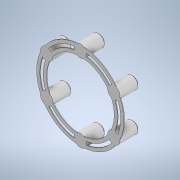
# Autodesk Inventor part: СкреплениеКатков
Saved by Autodesk Inventor 2020 (Build 240168000, 168)
## iProperties
Created: 2021-03-14
Part Number: СкреплениеКатков
Material: Типовые
Document SubType Name: Modeling
Designer: I_Love_U_Bogdan
Density: 1 g/cm^3
Appearance: По умолчанию
Author: I_Love_U_Bogdan
Autodesk Inventor part; units mm, degrees
ref_plane "YZ Plane" through (0, 0, 0) normal (1, 0, 0) x (0, 1, 0)
ref_plane "XZ Plane" through (0, 0, 0) normal (0, 1, 0) x (-1, 0, 0)
ref_plane "XY Plane" through (0, 0, 0) normal (0, 0, 1) x (1, 0, 0)
sketch "Эскиз1" plane through (0, 0, 0) normal (0, 0, 1) x (1, 0, 0)
  circle A0 centre (10.3923, 6) radius 2 projected
  circle A1 centre (10.3923, -6) radius 2 projected
  circle A2 centre (0, -12) radius 2 projected
  circle A3 centre (-10.3923, -6) radius 2 projected
  circle A4 centre (0, 0) radius 4 projected
  arc A5 (4.659, 13.202) -> (0, 14) centre (0, 0) ccw projected
  circle A6 centre (0, 12) radius 2 projected
  arc A7 (0, 14) -> (-4.659, 13.202) centre (0, 0) ccw projected
  arc A8 (-3.5064, 12.0732) -> (-4.659, 13.202) centre (-6.1045, 10.5732) ccw projected
  line L0 (-3.5064, 12.0732) -> (-2.63, 7.3847) projected
  arc A9 (-5.0804, 5.97) -> (-2.63, 7.3847) centre (-4.1045, 7.1091) ccw projected
  line L1 (-5.0804, 5.97) -> (-8.7025, 9.0732) projected
  arc A10 (-9.1038, 10.6358) -> (-8.7025, 9.0732) centre (-6.1045, 10.5732) ccw projected
  arc A11 (-9.1038, 10.6358) -> (-12.1244, 7) centre (0, 0) ccw projected
  circle A12 centre (-10.3923, 6) radius 2 projected
  arc A13 (-12.1244, 7) -> (-13.7628, 2.5662) centre (0, 0) ccw projected
  arc A14 (-12.2089, 3) -> (-13.7628, 2.5662) centre (-12.2089, 0) ccw projected
  line L2 (-12.2089, 3) -> (-7.7104, 1.4147) projected
  arc A15 (-7.7104, -1.4147) -> (-7.7104, 1.4147) centre (-8.2089, 0) ccw projected
  line L3 (-7.7104, -1.4147) -> (-12.2089, -3) projected
  arc A16 (-13.7628, -2.5662) -> (-12.2089, -3) centre (-12.2089, 0) ccw projected
  arc A17 (-13.7628, -2.5662) -> (-12.1244, -7) centre (0, 0) ccw projected
  circle A18 centre (-10.3923, -6) radius 2 projected
  arc A19 (-12.1244, -7) -> (-9.1038, -10.6358) centre (0, 0) ccw projected
  arc A20 (-8.7025, -9.0732) -> (-9.1038, -10.6358) centre (-6.1045, -10.5732) ccw projected
  line L4 (-8.7025, -9.0732) -> (-5.0804, -5.97) projected
  arc A21 (-2.63, -7.3847) -> (-5.0804, -5.97) centre (-4.1045, -7.1091) ccw projected
  line L5 (-2.63, -7.3847) -> (-3.5064, -12.0732) projected
  arc A22 (-4.659, -13.202) -> (-3.5064, -12.0732) centre (-6.1045, -10.5732) ccw projected
  arc A23 (-4.659, -13.202) -> (0, -14) centre (0, 0) ccw projected
  circle A24 centre (0, -12) radius 2 projected
  arc A25 (0, -14) -> (4.659, -13.202) centre (0, 0) ccw projected
  arc A26 (3.5064, -12.0732) -> (4.659, -13.202) centre (6.1045, -10.5732) ccw projected
  line L6 (3.5064, -12.0732) -> (2.63, -7.3847) projected
  arc A27 (5.0804, -5.97) -> (2.63, -7.3847) centre (4.1045, -7.1091) ccw projected
  line L7 (5.0804, -5.97) -> (8.7025, -9.0732) projected
  arc A28 (9.1038, -10.6358) -> (8.7025, -9.0732) centre (6.1045, -10.5732) ccw projected
  arc A29 (9.1038, -10.6358) -> (12.1244, -7) centre (0, 0) ccw projected
  circle A30 centre (10.3923, -6) radius 2 projected
  arc A31 (12.1244, -7) -> (13.7628, -2.5662) centre (0, 0) ccw projected
  arc A32 (12.2089, -3) -> (13.7628, -2.5662) centre (12.2089, 0) ccw projected
  line L8 (12.2089, -3) -> (7.7104, -1.4147) projected
  arc A33 (7.7104, 1.4147) -> (7.7104, -1.4147) centre (8.2089, 0) ccw projected
  line L9 (7.7104, 1.4147) -> (12.2089, 3) projected
  arc A34 (13.7628, 2.5662) -> (12.2089, 3) centre (12.2089, 0) ccw projected
  arc A35 (13.7628, 2.5662) -> (12.1244, 7) centre (0, 0) ccw projected
  circle A36 centre (10.3923, 6) radius 2 projected
  arc A37 (12.1244, 7) -> (9.1038, 10.6358) centre (0, 0) ccw projected
  arc A38 (8.7025, 9.0732) -> (9.1038, 10.6358) centre (6.1045, 10.5732) ccw projected
  line L10 (8.7025, 9.0732) -> (5.0804, 5.97) projected
  arc A39 (2.63, 7.3847) -> (5.0804, 5.97) centre (4.1045, 7.1091) ccw projected
  line L11 (2.63, 7.3847) -> (3.5064, 12.0732) projected
  arc A40 (4.659, 13.202) -> (3.5064, 12.0732) centre (6.1045, 10.5732) ccw projected
  circle A41 centre (10.3923, 6) radius 1.9
  circle A42 centre (0, 12) radius 1.9
  circle A43 centre (-10.3923, 6) radius 1.9
  circle A44 centre (-10.3923, -6) radius 1.9
  circle A45 centre (0, -12) radius 1.9
  circle A46 centre (10.3923, -6) radius 1.9
  point P0 (0, 0)
  dimension "d0" = 0.1
  dimension "d3" = 360
  constraints: 6 centre point, 3 vertical alignment, 20 other
extrude "Выдавливание1" add sketch "Эскиз1" along normal blind 2 and the other way blind 4 contours A41 | A42 | A43 | A44 | A45 | A46
sketch "Эскиз2" plane through (10.3923, 6, 2) normal (0, 0, 1) x (1, 0, 0)
  circle A0 centre (0, 0) radius 1.9 projected
  circle A1 centre (0, 0) radius 1.9 projected
  circle A2 centre (-10.3923, -6) radius 12
  circle A3 centre (-10.3923, -6) radius 10.5
  circle A4 centre (-10.3923, -6) radius 13.5
  circle A5 centre (-10.3923, -6) radius 12.5
  circle A6 centre (-10.3923, -6) radius 11.5
  point P0 (-0.8034, -1.7218)
  point P1 (-1.8928, 0.1651)
  point P2 (-0.621, 1.7956)
  point P3 (-1.4487, 1.2293)
  point P4 (0.3402, -1.8693)
  point P5 (1.2446, -1.4356)
  dimension "d9" = 1.5
  dimension "d12" = 1.5
  dimension "d13" = 0.5
  dimension "d14" = 0.5
  constraints: 4 centre point, 1 coincident, 3 other
extrude "Выдавливание2" add sketch "Эскиз2" against normal blind 0.2 contours A4 A0 A5 | A0 A5 A4 | A5 A0 A2 | A2 A0 A6 | A6 A0 A3 | A0 A3 A6 | A3 A0 picked at (0.2342, -0.105) picked at (-0.0588, -0.2643) picked at (-1.3755, -0.8832)
chamfer "Фаска1" distance 0.5 angle 45 6 edges at (8.4923, 6, -4) (-1.9, 12, -4) (8.4923, -6, -4) (-1.9, -12, -4) (-12.2923, -6, -4) (-12.2923, 6, -4)
